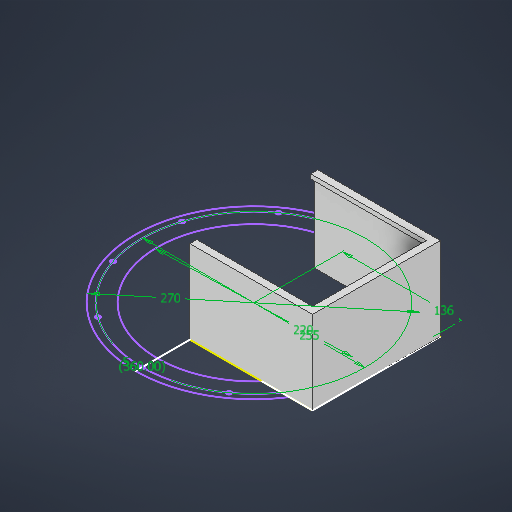
# Autodesk Inventor part: Galvo Housing-01
Saved by Autodesk Inventor 2025 (Build 290162000, 162)
## iProperties
Created: 2024-06-12
Part Number: Galvo Housing-01
Material: Generic
Document SubType Name: Modeling
Designer: mayhe
Density: 1 g/cm^3
Appearance: Default
Author: mayhe
Autodesk Inventor part; units mm, degrees
ref_plane "YZ Plane" through (0, 0, 0) normal (1, 0, 0) x (0, 1, 0)
ref_plane "XZ Plane" through (0, 0, 0) normal (0, 1, 0) x (-1, 0, 0)
ref_plane "XY Plane" through (0, 0, 0) normal (0, 0, 1) x (1, 0, 0)
sketch "Sketch4" plane through (0, 0, 0) normal (0, 1, 0) x (-1, 0, 0)
  line L0 (-70, 73) -> (70, 73)
  line L1 (70, -73) -> (-70, -73)
  line L2 (-70, -73) -> (-70, 73)
  line L3 (-66, -69) -> (70, -69)
  line L4 (70, 69) -> (-66, 69)
  line L5 (-66, 69) -> (-66, -69)
  line L6 (70, 73) -> (70, 69)
  line L7 (70, -69) -> (70, -73)
  point P0 (0, 0)
  point P1 (-66, 65)
  dimension "Housing_Length" = 140
  dimension "Housing_Width" = 146
  dimension "d15" = 4
  dimension "d36" = 136
  dimension "d37" = 138
  constraints: 16 end point, 4 parallel, 2 perpendicular, 1 horizontal
  measures "Housing_Length" distance of L1.start L1.end
  measures "Housing_Width" distance of L0.end L1.start
  measures "d15" distance between parallel lines of L1 L3
  measures "d36" distance of L3.start L3.end
  measures "d37" distance of L4.end L3.start
extrude "Extrusion4" add sketch "Sketch4" along normal blind 95
sketch "Sketch6" plane through (0, 95, 0) normal (0, 1, 0) x (1, 0, 0)
  line L0 (70, 73) -> (-70, 73) projected
  line L1 (-70, -69) -> (-70, -73) projected
  line L2 (70, 73) -> (-70, 73)
  line L3 (-70, 73) -> (-70, -73)
  line L4 (-70, -73) -> (70, -73)
  line L5 (70, -73) -> (70, 73)
  line L6 (62, -65) -> (-70, -65)
  line L7 (-70, 65) -> (62, 65)
  line L8 (62, 65) -> (62, -65)
  point P0 (0, 0)
  dimension "Lip_Width" = 8
  constraints: 14 end point, 3 parallel, 2 point on line, 1 horizontal, 1 perpendicular
  measures "Lip_Width" distance between parallel lines of L4 L6
extrude "Extrusion5" add sketch "Sketch6" against normal blind 5 contours L5 L4 L1 L3 L6 L8 L7 L0
sketch "Sketch10" plane through (0, 0, 0) normal (0, -1, 0) x (1, 0, 0)
  line L0 (66, -69) -> (66, 69) projected
  circle A0 centre (-70, 0) radius 135
  circle A1 centre (-70, 0) radius 110
  line L1 (-70, 73) -> (70, 73) projected
  line L2 (12.2861, 73) -> (70, 73)
  line L3 (70, -73) -> (-70, -73) projected
  line L4 (70, 73) -> (70, -73)
  line L5 (70, -73) -> (12.2861, -73)
  circle A2 centre (-70, 0) radius 127.5
  line L6 (-70, 0) -> (-70, 135)
  circle A3 centre (-70, 127.5) radius 2.5
  circle A4 centre (-144.9426, 103.1497) radius 2.5
  circle A5 centre (-191.2597, 39.3997) radius 2.5
  circle A6 centre (-191.2597, -39.3997) radius 2.5
  circle A7 centre (-144.9426, -103.1497) radius 2.5
  circle A8 centre (-70, -127.5) radius 2.5
  circle A9 centre (4.9426, -103.1497) radius 2.5
  circle A10 centre (51.2597, -39.3997) radius 2.5
  circle A11 centre (51.2597, 39.3997) radius 2.5
  circle A12 centre (4.9426, 103.1497) radius 2.5
  point P0 (0, 0)
  dimension "d52" = 270
  dimension "d57" = 255
  dimension "d53" = 136
  dimension "d54" = 220
  dimension "d58" = 5
  dimension "d61" = 360
  constraints: 11 centre point, 8 end point, 2 coincident, 2 point on circle, 2 point on line, 2 vertical alignment, 1 horizontal, 1 perpendicular, 1 vertical, 25 other
  measures "d53" distance from line of L0 point (-70, 0)
  measures "d54" diameter of A1
  measures "d58" diameter of A3
extrude "Extrusion9" add sketch "Sketch10" against normal blind 1 contours A0 L3 A2 A10 A11 L1 | A0 L1 L4 L3 | A2 A11 A10 L3 A1 L1
body "Solid2"
